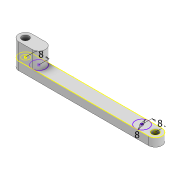
# Autodesk Inventor part: Part_4
Saved by Autodesk Inventor 2022 (Build 260153000, 153)
## iProperties
Created: 2022-04-21
Part Number: Part_4
Material: Generic
Document SubType Name: Modeling
Designer: dell
Density: 1 g/cm^3
Appearance: Default
Author: dell
Autodesk Inventor part; units mm, degrees
ref_plane "YZ Plane" through (0, 0, 0) normal (1, 0, 0) x (0, 1, 0)
ref_plane "XZ Plane" through (0, 0, 0) normal (0, 1, 0) x (-1, 0, 0)
ref_plane "XY Plane" through (0, 0, 0) normal (0, 0, 1) x (1, 0, 0)
sketch "Sketch1" plane through (0, 0, 0) normal (0, 1, 0) x (-1, 0, 0)
  line L0 (0, 0) -> (-77.789, 0) construction
  line L1 (0, 4) -> (-77.789, 4)
  line L2 (-77.789, -4) -> (0, -4)
  arc A0 (0, -4) -> (0, 4) centre (0, 0) ccw
  arc A1 (-77.789, 4) -> (-77.789, -4) centre (-77.789, 0) ccw
  circle A2 centre (0, 0) radius 2.1
  circle A3 centre (-77.789, 0) radius 2.1
  point P0 (-38.8945, 0)
  dimension "d0" = 77.789
  dimension "d1" = 8
  dimension "d2" = 4.2
  dimension "d10" = 4.2
  constraints: 8 end point, 4 centre point, 4 point on circle, 4 tangent, 2 coincident, 1 horizontal, 1 midpoint, 1 parallel
  measures "d0" distance of L0.end L0.start
  measures "d1" distance between parallel lines of L1 L2
  measures "d2" diameter of A2
  measures "d10" diameter of A3
extrude "Extrusion1" add sketch "Sketch1" along normal blind 5
sketch "Sketch2" plane through (0, 5, 0) normal (0, 1, 0) x (1, 0, 0)
  arc A0 (77.789, -4) -> (77.789, 4) centre (77.789, 0) ccw projected
  line L0 (77.789, 4) -> (0, 4) projected
  arc A1 (0, 4) -> (0, -4) centre (0, 0) ccw projected
  line L1 (0, -4) -> (77.789, -4) projected
  circle A2 centre (77.789, 0) radius 2.1 projected
  circle A3 centre (0, 0) radius 2.1 projected
  circle A4 centre (8, 0) radius 4
  line L2 (0, -4) -> (77.789, -4) projected
  circle A5 centre (69.789, 0) radius 4
  point P0 (69.789, -4)
  point P1 (69.789, 4)
  point P2 (8, -4)
  point P3 (8, 4)
  dimension "d11" = 8
  dimension "d12" = 8
  dimension "d13" = 8
  constraints: 2 centre point, 1 tangent
  measures "d11" distance of point (0, 0) A4.centre
  measures "d12" diameter of A5
  measures "d13" distance of A0.centre A5.centre
extrude "Extrusion2" add sketch "Sketch2" along normal blind 10 contours L1 A1 L0 A4 | A4
body "Solid1"
